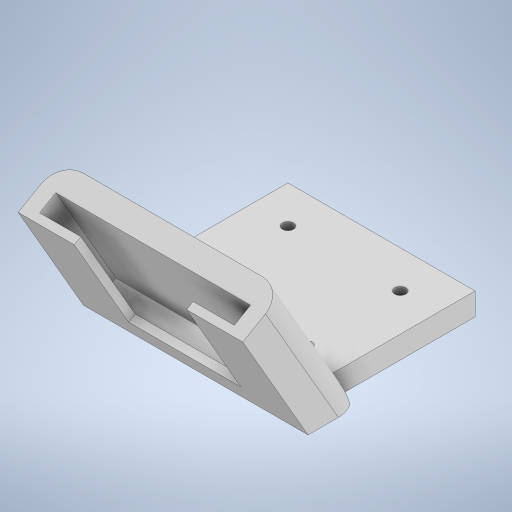
# Autodesk Inventor part: camera-mount
Saved by Autodesk Inventor 2024 (Build 280153000, 153)
## iProperties
Created: 2023-07-31
Part Number: camera-mount
Material: Generic
Document SubType Name: Modeling
Designer: cedri
Density: 1 g/cm^3
Appearance: Default
Author: cedri
Autodesk Inventor part; units mm, degrees
ref_plane "YZ Plane" through (0, 0, 0) normal (1, 0, 0) x (0, 1, 0)
ref_plane "XZ Plane" through (0, 0, 0) normal (0, 1, 0) x (-1, 0, 0)
ref_plane "XY Plane" through (0, 0, 0) normal (0, 0, 1) x (1, 0, 0)
sketch "Sketch1" plane through (0, 0, 0) normal (0, 1, 0) x (-1, 0, 0)
  line L0 (12.5, 11.25) -> (-12.5, 11.25)
  line L1 (-12.5, 11.25) -> (-12.5, -11.25)
  line L2 (-12.5, -11.25) -> (12.5, -11.25)
  line L3 (12.5, -11.25) -> (12.5, 11.25)
  line L4 (12.5, 11.25) -> (-12.5, -11.25) construction
  line L5 (-12.5, 11.25) -> (12.5, -11.25) construction
  line L6 (7.5, 6.25) -> (-7.5, 6.25) construction
  line L7 (-7.5, 6.25) -> (-7.5, -6.25) construction
  line L8 (-7.5, -6.25) -> (7.5, -6.25) construction
  line L9 (7.5, -6.25) -> (7.5, 6.25) construction
  line L10 (7.5, 6.25) -> (-7.5, -6.25) construction
  line L11 (-7.5, 6.25) -> (7.5, -6.25) construction
  circle A0 centre (7.5, -6.25) radius 0.75
  circle A1 centre (-7.5, -6.25) radius 0.75
  circle A2 centre (-7.5, 6.25) radius 0.75
  circle A3 centre (7.5, 6.25) radius 0.75
  point P0 (0, 0)
  dimension "d0" = 12.5
  dimension "d1" = 15
  dimension "d2" = 5
  dimension "d3" = 5
  dimension "d4" = 1.5
  dimension "d5" = 1.5
  dimension "d6" = 1.5
  dimension "d7" = 1.5
  constraints: 24 end point, 4 centre point, 4 coincident, 4 midpoint, 4 parallel, 2 horizontal, 2 perpendicular
  measures "d0" distance of L6.end L7.end
  measures "d1" distance of L7.end L8.end
  measures "d2" horizontal distance of L1.end L7.end
  measures "d3" horizontal distance of L1.end L7.end
  measures "d4" diameter of A0
  measures "d5" diameter of A1
  measures "d6" diameter of A2
  measures "d7" diameter of A3
extrude "Extrusion1" add sketch "Sketch1" along normal blind 3
ref_plane "Work Plane1" through (-12.5, 3, 11.25) normal (0, -0.5, 0.8660254) x (1, 0, 0)
sketch "Sketch2" plane through (-12.5, 3, 11.25) normal (0, -0.5, 0.8660254) x (1, 0, 0)
  line L0 (0, -11.25) -> (0, 0) construction
  line L1 (25, 0) -> (25, -11.25) construction
  line L2 (0, 0) -> (25, 0) construction
  line L3 (-2.5, 16) -> (27.5, 16)
  line L4 (27.5, 16) -> (27.5, -3)
  line L5 (27.5, -3) -> (-2.5, -3)
  line L6 (-2.5, -3) -> (-2.5, 16)
  line L7 (-2.5, 16) -> (27.5, -3) construction
  line L8 (27.5, 16) -> (-2.5, -3) construction
  point P0 (12.5, -8.2231)
  point P1 (12.5, 6.5)
  point P2 (12.5, 0)
  dimension "d11" = 19
  dimension "d12" = 16
  dimension "d13" = 30
  constraints: 14 end point, 3 midpoint, 2 horizontal, 2 parallel, 1 perpendicular, 1 vertical alignment
  measures "d11" distance of L3.end L4.end
  measures "d12" distance between parallel lines of L3 L2
  measures "d13" distance of L3.start L3.end
extrude "Extrusion2" add sketch "Sketch2" against normal blind 3
sketch "Sketch3" plane through (-12.5, 3, 11.25) normal (0, -0.5, 0.8660254) x (1, 0, 0)
  line L0 (0, 0) -> (25, 0) construction
  line L1 (-0.5, 0) -> (25.5, 0) construction
  line L2 (25.5, 0) -> (25.5, 16) construction
  line L3 (25.5, 16) -> (-0.5, 16) construction
  line L4 (-0.5, 16) -> (-0.5, 0) construction
  line L5 (-0.5, 0) -> (25.5, 16) construction
  line L6 (25.5, 0) -> (-0.5, 16) construction
  line L7 (-2.5, -3) -> (-2.5, 16) construction
  line L8 (-0.5, 16) -> (-2.5, 16)
  line L9 (-2.5, 16) -> (-2.5, 0)
  line L10 (-2.5, 0) -> (-0.5, 0)
  line L11 (-0.5, 0) -> (-0.5, 16)
  line L12 (27.5, 16) -> (27.5, -3) construction
  line L13 (25.5, 16) -> (27.5, 16)
  line L14 (27.5, 16) -> (27.5, 0)
  line L15 (27.5, 0) -> (25.5, 0)
  line L16 (25.5, 0) -> (25.5, 16)
  line L17 (-2.5, 0) -> (27.5, 0)
  line L18 (27.5, 0) -> (27.5, -2)
  line L19 (27.5, -2) -> (-2.5, -2)
  line L20 (-2.5, -2) -> (-2.5, 0)
  point P0 (12.5, -8.2231)
  point P1 (12.5, 8)
  point P2 (12.5, 0)
  point P3 (-0.5, 0)
  dimension "d16" = 16
  dimension "d17" = 26
  dimension "d18" = 2
  constraints: 36 end point, 8 parallel, 4 horizontal, 4 perpendicular, 3 collinear, 3 midpoint, 3 point on line, 1 vertical alignment
  measures "d16" distance of L1.end L2.end
  measures "d17" distance of L2.end L3.end
  measures "d18" distance between parallel lines of L17 L19
extrude "Extrusion3" add sketch "Sketch3" along normal blind 2.5
sketch "Sketch4" plane through (-12.5, 1.75, 13.4151) normal (0, -0.5, 0.8660254) x (1, 0, 0)
  line L0 (-2.5, 16) -> (-2.5, -2) projected
  line L1 (-2.5, -2) -> (27.5, -2) projected
  line L2 (27.5, -2) -> (27.5, 16) projected
  line L3 (27.5, 16) -> (25.5, 16) construction
  line L4 (-0.5, 16) -> (-2.5, 16) construction
  line L5 (-2.5, -2) -> (27.5, -2) construction
  line L6 (27.5, -2) -> (27.5, 16) construction
  line L7 (27.5, 16) -> (-2.5, 16)
  line L8 (-2.5, 16) -> (-2.5, -2) construction
  line L9 (5, 1.5) -> (20, 1.5)
  line L10 (20, 1.5) -> (20, 16)
  line L11 (20, 16) -> (5, 16)
  line L12 (5, 16) -> (5, 1.5)
  line L13 (5, 1.5) -> (20, 16) construction
  line L14 (20, 1.5) -> (5, 16) construction
  point P0 (12.5, -8.2231)
  point P1 (12.5, 8.75)
  point P2 (12.5, 16)
  point P3 (20, 16)
  dimension "d21" = 15
  dimension "d23" = 3.5
  constraints: 20 end point, 4 parallel, 3 midpoint, 2 horizontal, 2 perpendicular, 1 collinear, 1 vertical alignment
  measures "d21" distance of L10.end L11.end
  measures "d23" distance between parallel lines of L9 L1
extrude "Extrusion4" add sketch "Sketch4" along normal blind 1 contours L7 L12 L9 L10 L2 L1 L0
sketch "Sketch5" plane through (12.5, 1.2679, 10.25) normal (0, -0.8660254, -0.5) x (1, 0, 0)
  line L0 (2.5, 0) -> (2.5, 3.5) projected
  line L1 (0, 0) -> (0, 1.1547) projected
  line L2 (2.5, 0) -> (0, 0) projected
  line L3 (-27.5, 3.5) -> (2.5, 3.5) projected
  line L4 (0, 1.1547) -> (-25, 1.1547) projected
  line L5 (-25, 0) -> (-27.5, 0) projected
  line L6 (-27.5, 0) -> (-27.5, 3.5) projected
  line L7 (-25, 1.1547) -> (-25, 0) projected
  point P0 (-12.5, -8.2428)
extrude "Extrusion5" add sketch "Sketch5" along normal blind 1
sketch "Sketch6" plane through (12.5, 1.9019, 7.1519) normal (0, -0.8660254, -0.5) x (1, 0, 0)
  line L0 (2.5, 0) -> (0, 0) projected
  line L1 (-25, 4.1547) -> (0, 4.1547) projected
  line L2 (-25, 0) -> (-27.5, 0) projected
  line L3 (2.5, 0) -> (-27.5, 0)
  line L4 (-27.5, 0) -> (-27.5, 4.1547)
  line L5 (-27.5, 4.1547) -> (2.5, 4.1547)
  line L6 (2.5, 4.1547) -> (2.5, 0)
  point P0 (-12.5, -5.2428)
  constraints: 8 end point, 2 parallel, 1 horizontal, 1 perpendicular, 1 point on line
sketch3d "3D Sketch1"
  line L0 (12.5, 3, -11.25) -> (12.5, 0, -11.25)
sweep "Sweep1" add profiles "Sketch6" path "3D Sketch1"
sketch "Sketch7" plane through (12.5, 0, -11.25) normal (0, 0, -1) x (-1, 0, 0)
  line L0 (-2.5, 0) -> (27.5, 0)
  line L1 (27.5, 0) -> (27.5, -3.1754)
  line L2 (27.5, -3.1754) -> (-2.5, -3.1754)
  line L3 (-2.5, -3.1754) -> (-2.5, 0)
  line L4 (0, 0) -> (25, 0) projected
  line L5 (27.5, 1.9019) -> (27.5, -1.0981) projected
  line L6 (-2.5, 1.9019) -> (-2.5, -1.0981) projected
  line L7 (-2.5, -3.1754) -> (27.5, -3.1754) projected
  point P0 (12.5, 0)
  constraints: 8 end point, 4 collinear, 2 parallel, 1 horizontal, 1 perpendicular
extrude "Extrusion6" cut sketch "Sketch7" against normal through all
fillet "Fillet1" radius 3 2 edges at (15, 10.1292, 11.9019) (-15, 10.1292, 11.9019)
equation "\"d5\" = d4"
equation "\"d6\" = d4"
equation "\"d7\" = d4"
body "Solid1"
